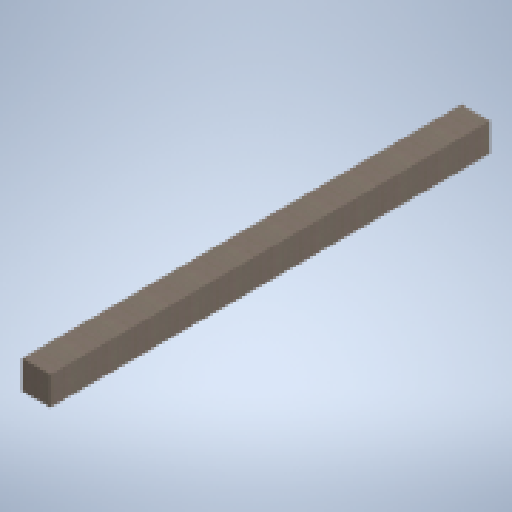
# Autodesk Inventor part: BaseLarge
Saved by Autodesk Inventor 2025.2 (Build 292293000, 293)
## iProperties
Created: 2025-03-06
Part Number: BaseLarge
Material: Wood (Walnut)
Document SubType Name: Modeling
Designer: baolo
Density: 0.55 g/cm^3
Appearance: Walnut
Mass: 94.6 g
Surface Area: 352 cm^2
Volume: 172 cm^3
Author: baolo
Autodesk Inventor part; units mm, degrees
ref_plane "YZ Plane" through (0, 0, 0) normal (1, 0, 0) x (0, 1, 0)
ref_plane "XZ Plane" through (0, 0, 0) normal (0, 1, 0) x (-1, 0, 0)
ref_plane "XY Plane" through (0, 0, 0) normal (0, 0, 1) x (1, 0, 0)
sketch "Sketch1" plane through (0, 0, 0) normal (0, 1, 0) x (-1, 0, 0)
  line L0 (8.7312, 135) -> (-8.7313, 135)
  line L1 (-8.7313, 135) -> (-8.7313, -135)
  line L2 (-8.7313, -135) -> (8.7312, -135)
  line L3 (8.7312, -135) -> (8.7312, 135)
  line L4 (8.7312, 135) -> (-8.7313, -135) construction
  line L5 (-8.7313, 135) -> (8.7312, -135) construction
  point P0 (0, 0)
  dimension "d0" = 270
  dimension "d1" = 17.4625
  constraints: 12 end point, 2 midpoint, 2 parallel, 1 horizontal, 1 perpendicular
  measures "d0" distance between parallel lines of L2 L0
  measures "d1" distance between parallel lines of L1 L3
extrude "Extrusion1" add sketch "Sketch1" along normal mid plane 17.4625
equation "\"StockSize\" = 38.1"
body "Solid1"
